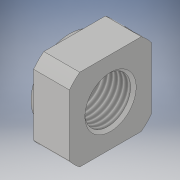
# Autodesk Inventor part: C-TFK10_n
Saved by Autodesk Inventor 2021 (Build 250183000, 183)
## iProperties
Created: 2023-03-01
Part Number: C-TFK10_n
Material: Generic
Catalog Web Link: www.cadenas.de
Description: C-TFK_n-Economy Support Units Fixed Side Round
Vendor: MISUMI
Document SubType Name: Modeling
Designer: psAdmin
Manufacturer: MISUMI
Mass: 1.3831 g
Surface Area: 10.7484 cm^2
Volume: 1.3831 cm^3
Density: 1 g/cm^3
Appearance: PSOLRGB-175-175-175
Category: PARTsolutions
Company: MISUMI
PSOL_IDENT_0: {$CADENAS_DATA/23d-libs/misumi/metric/09_ball_screws/c_tfk/c_tfk_nut.prj},161 {VTYP=3D},{NB=C-TFK10_
PSOL_IDENT_1: n},{LINA=C-TFK10},{NN=C-TFK_n},{DATE=14.09.2022 01:48:07},{GEOMDATE=16.11.2021 00:32:38},{VERSION=},
PSOL_IDENT_2: {LINEID=100},{WBVAR=SET},{WBNUMERIC=}  {NB=C-TFK10_n},{LINA=C-TFK10},{KT=DUMMY},{PN=C-TFK10},{TYPE=C
PSOL_IDENT_3: -TFK},{NO=10},{SET=},{DD=10},{L=27},{H=10},{F=17},{E=29.5},{D=34},{A=52},{PCD=42},{B=42},{L1=7.5},{T
PSOL_IDENT_4: 1=5.0},{DD1=4.5},{DD2=8.0},{LL=4.0},{M=M10x1.0},{T=16},{ACNM=M10x1.0},{M0=10},{ACNB=8.0},{ACNMM=M3},
PSOL_IDENT_5: {ACNMM3D=3},{ACNDD=15},{ACND=20.0},{ACNF=16},{SID=14.0},{N3=1.0},{N4=2.5},{PITCH=1.00}
NB: C-TFK10_n
NN: C-TFK_n
NT: Economy Support Units Fixed Side Round
NBSYN: $PN._n
LINA: C-TFK10
CATALOG: Misumi
PN: C-TFK10
NO: 10
SET: w/o SET
DD: 10
L: 27
H: 10
F: 17
E: 29.5
D: 34
A: 52
PCD: 42
B: 42
L1: 7.5
T1: 5
DD1: 4.5
DD2: 8
LL: 4
M: M10x1.0
T: 16
ACNM: M10x1.0
ACNB: 8
ACNMM: M3
ACNDD: 15
ACND: 20
ACNF: 16
SUPPLIER: MISUMI
ARTICLENO: C-TFK10_n
BOMINFO: C-TFK10
CREATOR: CADENAS GmbH
Title: C-TFK10
Author: Cadenas PARTsolutions
Comments: Economy Support Units Fixed Side Round
Autodesk Inventor part; units mm, degrees
sketch "Sketch_1" plane through (0, 0, 0) normal (1, 0, 0) x (0, 0, -1)
  line L0 (-8, 6) -> (-8, -6)
  arc A0 (-8, -6) -> (-6, -8) centre (0, 0) ccw
  line L1 (-6, -8) -> (6, -8)
  arc A1 (6, -8) -> (8, -6) centre (0, 0) ccw
  line L2 (8, -6) -> (8, 6)
  arc A2 (8, 6) -> (6, 8) centre (0, 0) ccw
  line L3 (6, 8) -> (-6, 8)
  arc A3 (-6, 8) -> (-8, 6) centre (0, 0) ccw
  constraints: 8 end point, 8 point on circle, 4 centre point
extrude "Extrusion1" add sketch "Sketch_1" along normal blind 7
sketch "Sketch_2" plane through (0, 0, 0) normal (0, 0, 1) x (1, 0, 0)
  line L0 (0, 0) -> (-1, 0)
  line L1 (-1, 0) -> (-1, 7.5)
  line L2 (-1, 7.5) -> (0, 7.5)
  line L3 (0, 7.5) -> (0, 0)
  line L4 (0, 0) -> (-1, 0)
  constraints: 10 end point
revolve "Revolution1" add sketch "Sketch_2" angle 360 about axis through (0, 0, 0) along (1, 0, 0)
sketch "Sketch_3" plane through (0, 0, 0) normal (0, 0, 1) x (1, 0, 0)
  line L0 (7, 0) -> (-1, 0)
  line L1 (-1, 0) -> (-1, 5)
  line L2 (-1, 5) -> (-0.4585, 4.4585)
  line L3 (-0.4585, 4.4585) -> (6.4585, 4.4585)
  line L4 (6.4585, 4.4585) -> (7, 5)
  line L5 (7, 5) -> (7, 0)
  line L6 (7, 0) -> (-1, 0)
  constraints: 14 end point
revolve "Revolution2" cut sketch "Sketch_3" angle 360 about axis through (7, 0, 0) along (1, 0, 0)
thread "Thread1" size "M10x1" class "6H" standard "ISO Metric profile" full length
sketch "Sketch_4" plane through (4.5, 0, 0) normal (1, 0, 0) x (0, 0, -1)
  line L0 (0, 0) -> (7.0711, 7.0711)
  line L1 (7.0711, 7.0711) -> (8.1317, 6.0104)
  line L2 (8.1317, 6.0104) -> (7.7492, 6.0104)
  line L3 (7.7492, 6.0104) -> (0.8694, -0.8694)
  line L4 (0.8694, -0.8694) -> (0, 0)
  line L5 (0, 0) -> (7.0711, 7.0711)
  constraints: 12 end point
revolve "Revolution3" cut sketch "Sketch_4" angle 360 about axis through (4.5, 0, 0) along (0, -0.7071068, 0.7071068)
thread "Thread2" size "M3x0.5" class "6H" standard "ISO Metric profile" full length
ref_plane "to_collar_XY" through (-1, 0, 0) normal (-1, 0, 0) x (0, -0.7071068, -0.7071068)
ref_plane "to_collar_YZ" through (-1, 0, 0) normal (0, -0.7071068, -0.7071068) x (0, -0.7071068, 0.7071068)
ref_plane "to_collar_ZX" through (-1, 0, 0) normal (0, -0.7071068, 0.7071068) x (-1, 0, 0)
body "Solid1"
